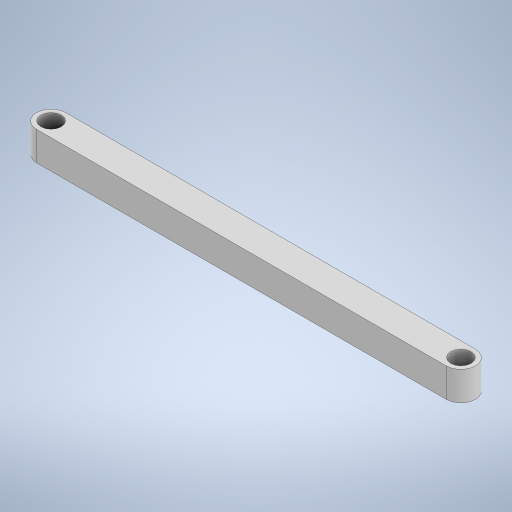
# Autodesk Inventor part: 4-bar intake (14.112) bar
Saved by Autodesk Inventor 2023 (Build 270158030, 158C)
## iProperties
Created: 2022-07-18
Part Number: 4-bar intake (14.112) bar
Material: Generic
Document SubType Name: Modeling
Designer: kt1040502
Density: 1 g/cm^3
Appearance: Default
Author: kt1040502
Autodesk Inventor part; units mm, degrees
ref_plane "YZ Plane" through (0, 0, 0) normal (1, 0, 0) x (0, 1, 0)
ref_plane "XZ Plane" through (0, 0, 0) normal (0, 1, 0) x (-1, 0, 0)
ref_plane "XY Plane" through (0, 0, 0) normal (0, 0, 1) x (1, 0, 0)
sketch "Sketch1" plane through (0, 0, 0) normal (0, 1, 0) x (-1, 0, 0)
  line L0 (0, 0) -> (-358.4448, 0)
  line L1 (0, 0) -> (-358.4448, 0) construction
  line L2 (0, 12.7) -> (-358.4448, 12.7)
  line L3 (-358.4448, -12.7) -> (0, -12.7)
  arc A0 (0, -12.7) -> (0, 12.7) centre (0, 0) ccw
  arc A1 (-358.4448, 12.7) -> (-358.4448, -12.7) centre (-358.4448, 0) ccw
  arc A2 (0, 12.7) -> (0, -12.7) centre (0, 0) ccw
  arc A3 (-358.4448, -12.7) -> (-358.4448, 12.7) centre (-358.4448, 0) ccw
  point P0 (-179.2224, 0)
  dimension "d0" = 358.4448
  dimension "d1" = 25.4
  constraints: 10 end point, 8 point on circle, 8 tangent, 4 centre point, 2 equal length, 2 point on line, 1 horizontal, 1 midpoint
  measures "d0" distance of L0.start L0.end
  measures "d1" diameter of A1
extrude "Extrusion1" add sketch "Sketch1" along normal blind 25.4
sketch "Sketch2" plane through (0, 25.4, 0) normal (0, 1, 0) x (1, 0, 0)
  arc A0 (0, 12.7) -> (0, -12.7) centre (0, 0) ccw projected
  circle A1 centre (0, 0) radius 8.89
  arc A2 (358.4448, -12.7) -> (358.4448, 12.7) centre (358.4448, 0) ccw projected
  circle A3 centre (358.4448, 0) radius 8.89
  dimension "d4" = 17.78
  dimension "d5" = 17.78
  constraints: 2 centre point, 2 coincident
  measures "d4" diameter of A1
  measures "d5" diameter of A3
extrude "Extrusion2" cut sketch "Sketch2" against normal blind 25.4
body "Solid1"
